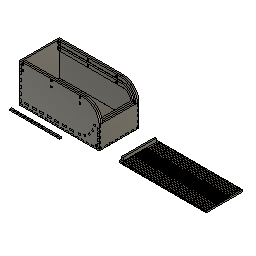
skuffa v30 (Autodesk Fusion 360 design; units mm, degrees)
Autodesk Fusion 360 part; units mm, degrees
note: some values were not read from the file. Chosen so that the rebuilt part matches the saved one: a direction. Set by a fixed rule: which sketch regions a step uses; which face or edge a step refers to.
(part 1 of 6)
sketch "Sketch1" plane through (0, 0, 0) normal (0, 0, 1) x (1, 0, 0)
  line L0 (2.6723, -62.3358) -> (29.1306, -62.3358)
  line L1 (29.1306, -62.3358) -> (29.1306, -59.69)
  line L2 (29.1306, -59.69) -> (2.6723, -59.69)
  line L3 (2.6723, -59.69) -> (2.6723, -62.3358)
  line L4 (5.3181, -57.2294) -> (4.5508, -57.2294)
  spline S0 degree 3 poles (4.5508, -57.2294) (4.5244, -57.2294) (4.5508, -57.2558) (4.5508, -57.2294) knots 0 0 0 0 1 1 1 1
  line L5 (4.5508, -57.2294) -> (4.5508, -56.4885)
  spline S1 degree 3 poles (4.5508, -56.4885) (4.5508, -56.4621) (4.5244, -56.4885) (4.5508, -56.4885) knots 0 0 0 0 1 1 1 1
  line L6 (4.5508, -56.4885) -> (6.0854, -56.4885)
  spline S2 degree 3 poles (6.0854, -56.4885) (6.1119, -56.4885) (6.0854, -56.4621) (6.0854, -56.4885) knots 0 0 0 0 1 1 1 1
  line L7 (6.0854, -56.4885) -> (6.0854, -57.2294)
  spline S3 degree 3 poles (6.0854, -57.2294) (6.0854, -57.2558) (6.1119, -57.2294) (6.0854, -57.2294) knots 0 0 0 0 1 1 1 1
  line L8 (6.0854, -57.2294) -> (5.3181, -57.2294)
  line L9 (8.4931, -57.2294) -> (7.7258, -57.2294)
  spline S4 degree 3 poles (7.7258, -57.2294) (7.6994, -57.2294) (7.7258, -57.2558) (7.7258, -57.2294) knots 0 0 0 0 1 1 1 1
  line L10 (7.7258, -57.2294) -> (7.7258, -56.4885)
  spline S5 degree 3 poles (7.7258, -56.4885) (7.7258, -56.4621) (7.6994, -56.4885) (7.7258, -56.4885) knots 0 0 0 0 1 1 1 1
  line L11 (7.7258, -56.4885) -> (9.2604, -56.4885)
  spline S6 degree 3 poles (9.2604, -56.4885) (9.2869, -56.4885) (9.2604, -56.4621) (9.2604, -56.4885) knots 0 0 0 0 1 1 1 1
  line L12 (9.2604, -56.4885) -> (9.2604, -57.2294)
  spline S7 degree 3 poles (9.2604, -57.2294) (9.2604, -57.2558) (9.2869, -57.2294) (9.2604, -57.2294) knots 0 0 0 0 1 1 1 1
  line L13 (9.2604, -57.2294) -> (8.4931, -57.2294)
  line L14 (11.6681, -57.2294) -> (10.9008, -57.2294)
  spline S8 degree 3 poles (10.9008, -57.2294) (10.8744, -57.2294) (10.9008, -57.2558) (10.9008, -57.2294) knots 0 0 0 0 1 1 1 1
  line L15 (10.9008, -57.2294) -> (10.9008, -56.4885)
  spline S9 degree 3 poles (10.9008, -56.4885) (10.9008, -56.4621) (10.8744, -56.4885) (10.9008, -56.4885) knots 0 0 0 0 1 1 1 1
  line L16 (10.9008, -56.4885) -> (12.4354, -56.4885)
  spline S10 degree 3 poles (12.4354, -56.4885) (12.4619, -56.4885) (12.4354, -56.4621) (12.4354, -56.4885) knots 0 0 0 0 1 1 1 1
  line L17 (12.4354, -56.4885) -> (12.4354, -57.2294)
  spline S11 degree 3 poles (12.4354, -57.2294) (12.4354, -57.2558) (12.4619, -57.2294) (12.4354, -57.2294) knots 0 0 0 0 1 1 1 1
  line L18 (12.4354, -57.2294) -> (11.6681, -57.2294)
  line L19 (14.8431, -57.2294) -> (14.0758, -57.2294)
  spline S12 degree 3 poles (14.0758, -57.2294) (14.0494, -57.2294) (14.0758, -57.2558) (14.0758, -57.2294) knots 0 0 0 0 1 1 1 1
  line L20 (14.0758, -57.2294) -> (14.0758, -56.4885)
  spline S13 degree 3 poles (14.0758, -56.4885) (14.0758, -56.4621) (14.0494, -56.4885) (14.0758, -56.4885) knots 0 0 0 0 1 1 1 1
  line L21 (14.0758, -56.4885) -> (15.6104, -56.4885)
  spline S14 degree 3 poles (15.6104, -56.4885) (15.6369, -56.4885) (15.6104, -56.4621) (15.6104, -56.4885) knots 0 0 0 0 1 1 1 1
  line L22 (15.6104, -56.4885) -> (15.6104, -57.2294)
  spline S15 degree 3 poles (15.6104, -57.2294) (15.6104, -57.2558) (15.6369, -57.2294) (15.6104, -57.2294) knots 0 0 0 0 1 1 1 1
  line L23 (15.6104, -57.2294) -> (14.8431, -57.2294)
  line L24 (18.0181, -57.2294) -> (17.2508, -57.2294)
  spline S16 degree 3 poles (17.2508, -57.2294) (17.2244, -57.2294) (17.2508, -57.2558) (17.2508, -57.2294) knots 0 0 0 0 1 1 1 1
  line L25 (17.2508, -57.2294) -> (17.2508, -56.4885)
  spline S17 degree 3 poles (17.2508, -56.4885) (17.2508, -56.4621) (17.2244, -56.4885) (17.2508, -56.4885) knots 0 0 0 0 1 1 1 1
  line L26 (17.2508, -56.4885) -> (18.7854, -56.4885)
  spline S18 degree 3 poles (18.7854, -56.4885) (18.8119, -56.4885) (18.7854, -56.4621) (18.7854, -56.4885) knots 0 0 0 0 1 1 1 1
  line L27 (18.7854, -56.4885) -> (18.7854, -57.2294)
  spline S19 degree 3 poles (18.7854, -57.2294) (18.7854, -57.2558) (18.8119, -57.2294) (18.7854, -57.2294) knots 0 0 0 0 1 1 1 1
  line L28 (18.7854, -57.2294) -> (18.0181, -57.2294)
  line L29 (21.1931, -57.2294) -> (20.4258, -57.2294)
  spline S20 degree 3 poles (20.4258, -57.2294) (20.3994, -57.2294) (20.4258, -57.2558) (20.4258, -57.2294) knots 0 0 0 0 1 1 1 1
  line L30 (20.4258, -57.2294) -> (20.4258, -56.4885)
  spline S21 degree 3 poles (20.4258, -56.4885) (20.4258, -56.4621) (20.3994, -56.4885) (20.4258, -56.4885) knots 0 0 0 0 1 1 1 1
  line L31 (20.4258, -56.4885) -> (21.9604, -56.4885)
  spline S22 degree 3 poles (21.9604, -56.4885) (21.9869, -56.4885) (21.9604, -56.4621) (21.9604, -56.4885) knots 0 0 0 0 1 1 1 1
  line L32 (21.9604, -56.4885) -> (21.9604, -57.2294)
  spline S23 degree 3 poles (21.9604, -57.2294) (21.9604, -57.2558) (21.9869, -57.2294) (21.9604, -57.2294) knots 0 0 0 0 1 1 1 1
  line L33 (21.9604, -57.2294) -> (21.1931, -57.2294)
  line L34 (24.3681, -57.2294) -> (23.6008, -57.2294)
  spline S24 degree 3 poles (23.6008, -57.2294) (23.5744, -57.2294) (23.6008, -57.2558) (23.6008, -57.2294) knots 0 0 0 0 1 1 1 1
  line L35 (23.6008, -57.2294) -> (23.6008, -56.4885)
  spline S25 degree 3 poles (23.6008, -56.4885) (23.6008, -56.4621) (23.5744, -56.4885) (23.6008, -56.4885) knots 0 0 0 0 1 1 1 1
  line L36 (23.6008, -56.4885) -> (25.1354, -56.4885)
  spline S26 degree 3 poles (25.1354, -56.4885) (25.1619, -56.4885) (25.1354, -56.4621) (25.1354, -56.4885) knots 0 0 0 0 1 1 1 1
  line L37 (25.1354, -56.4885) -> (25.1354, -57.2294)
  spline S27 degree 3 poles (25.1354, -57.2294) (25.1354, -57.2558) (25.1619, -57.2294) (25.1354, -57.2294) knots 0 0 0 0 1 1 1 1
  line L38 (25.1354, -57.2294) -> (24.3681, -57.2294)
  line L39 (27.5431, -57.2294) -> (26.7758, -57.2294)
  spline S28 degree 3 poles (26.7758, -57.2294) (26.7494, -57.2294) (26.7758, -57.2558) (26.7758, -57.2294) knots 0 0 0 0 1 1 1 1
  line L40 (26.7758, -57.2294) -> (26.7758, -56.4885)
  spline S29 degree 3 poles (26.7758, -56.4885) (26.7758, -56.4621) (26.7494, -56.4885) (26.7758, -56.4885) knots 0 0 0 0 1 1 1 1
  line L41 (26.7758, -56.4885) -> (28.3104, -56.4885)
  spline S30 degree 3 poles (28.3104, -56.4885) (28.3369, -56.4885) (28.3104, -56.4621) (28.3104, -56.4885) knots 0 0 0 0 1 1 1 1
  line L42 (28.3104, -56.4885) -> (28.3104, -57.2294)
  spline S31 degree 3 poles (28.3104, -57.2294) (28.3104, -57.2558) (28.3369, -57.2294) (28.3104, -57.2294) knots 0 0 0 0 1 1 1 1
  line L43 (28.3104, -57.2294) -> (27.5431, -57.2294)
  line L44 (30.7181, -57.2294) -> (29.9508, -57.2294)
  spline S32 degree 3 poles (29.9508, -57.2294) (29.9244, -57.2294) (29.9508, -57.2558) (29.9508, -57.2294) knots 0 0 0 0 1 1 1 1
  line L45 (29.9508, -57.2294) -> (29.9508, -56.4885)
  spline S33 degree 3 poles (29.9508, -56.4885) (29.9508, -56.4621) (29.9244, -56.4885) (29.9508, -56.4885) knots 0 0 0 0 1 1 1 1
  line L46 (29.9508, -56.4885) -> (31.4854, -56.4885)
  spline S34 degree 3 poles (31.4854, -56.4885) (31.5119, -56.4885) (31.4854, -56.4621) (31.4854, -56.4885) knots 0 0 0 0 1 1 1 1
  line L47 (31.4854, -56.4885) -> (31.4854, -57.2294)
  spline S35 degree 3 poles (31.4854, -57.2294) (31.4854, -57.2558) (31.5119, -57.2294) (31.4854, -57.2294) knots 0 0 0 0 1 1 1 1
  line L48 (31.4854, -57.2294) -> (30.7181, -57.2294)
  line L49 (34.9186, -56.6272) -> (34.1773, -56.8259)
  spline S36 degree 3 poles (34.1773, -56.8259) (34.1519, -56.8328) (34.1842, -56.8513) (34.1773, -56.8259) knots 0 0 0 0 1 1 1 1
  line L50 (34.1773, -56.8259) -> (33.9857, -56.1102)
  spline S37 degree 3 poles (33.9857, -56.1102) (33.9788, -56.0845) (33.9601, -56.1171) (33.9857, -56.1102) knots 0 0 0 0 1 1 1 1
  line L51 (33.9857, -56.1102) -> (35.4679, -55.713)
  spline S38 degree 3 poles (35.4679, -55.713) (35.4936, -55.7062) (35.461, -55.6874) (35.4679, -55.713) knots 0 0 0 0 1 1 1 1
  line L52 (35.4679, -55.713) -> (35.6597, -56.4287)
  spline S39 degree 3 poles (35.6597, -56.4287) (35.6666, -56.4541) (35.6851, -56.4219) (35.6597, -56.4287) knots 0 0 0 0 1 1 1 1
  line L53 (35.6597, -56.4287) -> (34.9186, -56.6272)
  line L54 (38.9861, -54.279) -> (38.4434, -54.8214)
  spline S40 degree 3 poles (38.4434, -54.8214) (38.4246, -54.8402) (38.4622, -54.8402) (38.4434, -54.8214) knots 0 0 0 0 1 1 1 1
  line L55 (38.4434, -54.8214) -> (37.9196, -54.2975)
  spline S41 degree 3 poles (37.9196, -54.2975) (37.9008, -54.279) (37.9008, -54.3163) (37.9196, -54.2975) knots 0 0 0 0 1 1 1 1
  line L56 (37.9196, -54.2975) -> (39.0046, -53.2125)
  spline S42 degree 3 poles (39.0046, -53.2125) (39.0234, -53.1937) (38.9861, -53.1937) (39.0046, -53.2125) knots 0 0 0 0 1 1 1 1
  line L57 (39.0046, -53.2125) -> (39.5285, -53.7363)
  spline S43 degree 3 poles (39.5285, -53.7363) (39.5473, -53.7551) (39.5473, -53.7176) (39.5285, -53.7363) knots 0 0 0 0 1 1 1 1
  line L58 (39.5285, -53.7363) -> (38.9861, -54.279)
  line L59 (41.3343, -50.2116) -> (41.1358, -50.9527)
  spline S44 degree 3 poles (41.1358, -50.9527) (41.1289, -50.9781) (41.1612, -50.9595) (41.1358, -50.9527) knots 0 0 0 0 1 1 1 1
  line L60 (41.1358, -50.9527) -> (40.4201, -50.7608)
  spline S45 degree 3 poles (40.4201, -50.7608) (40.3945, -50.754) (40.4133, -50.7865) (40.4201, -50.7608) knots 0 0 0 0 1 1 1 1
  line L61 (40.4201, -50.7608) -> (40.8173, -49.2786)
  spline S46 degree 3 poles (40.8173, -49.2786) (40.8242, -49.253) (40.7916, -49.2718) (40.8173, -49.2786) knots 0 0 0 0 1 1 1 1
  line L62 (40.8173, -49.2786) -> (41.533, -49.4702)
  spline S47 degree 3 poles (41.533, -49.4702) (41.5584, -49.4771) (41.5398, -49.4448) (41.533, -49.4702) knots 0 0 0 0 1 1 1 1
  line L63 (41.533, -49.4702) -> (41.3343, -50.2116)
  line L64 (41.9365, -45.2173) -> (41.9365, -45.9846)
  spline S48 degree 3 poles (41.9365, -45.9846) (41.9365, -46.011) (41.9629, -45.9846) (41.9365, -45.9846) knots 0 0 0 0 1 1 1 1
  line L65 (41.9365, -45.9846) -> (41.1956, -45.9846)
  spline S49 degree 3 poles (41.1956, -45.9846) (41.1692, -45.9846) (41.1956, -46.011) (41.1956, -45.9846) knots 0 0 0 0 1 1 1 1
  line L66 (41.1956, -45.9846) -> (41.1956, -44.45)
  spline S50 degree 3 poles (41.1956, -44.45) (41.1956, -44.4235) (41.1692, -44.45) (41.1956, -44.45) knots 0 0 0 0 1 1 1 1
  line L67 (41.1956, -44.45) -> (41.9365, -44.45)
  spline S51 degree 3 poles (41.9365, -44.45) (41.9629, -44.45) (41.9365, -44.4235) (41.9365, -44.45) knots 0 0 0 0 1 1 1 1
  line L68 (41.9365, -44.45) -> (41.9365, -45.2173)
  line L69 (3.466, -58.4465) -> (5.0271, -58.4465)
  spline S52 degree 3 poles (5.0271, -58.4465) (5.0535, -58.4465) (5.0271, -58.42) (5.0271, -58.4465) knots 0 0 0 0 1 1 1 1
  line L70 (5.0271, -58.4465) -> (5.0271, -59.2138)
  spline S53 degree 3 poles (5.0271, -59.2138) (5.0271, -59.2283) (5.039, -59.2402) (5.0535, -59.2402) knots 0 0 0 0 1 1 1 1
  line L71 (5.0535, -59.2402) -> (6.641, -59.2402)
  spline S54 degree 3 poles (6.641, -59.2402) (6.6556, -59.2402) (6.6675, -59.2283) (6.6675, -59.2138) knots 0 0 0 0 1 1 1 1
  line L72 (6.6675, -59.2138) -> (6.6675, -58.4465)
  spline S55 degree 3 poles (6.6675, -58.4465) (6.6675, -58.42) (6.641, -58.4465) (6.6675, -58.4465) knots 0 0 0 0 1 1 1 1
  line L73 (6.6675, -58.4465) -> (8.2021, -58.4465)
  spline S56 degree 3 poles (8.2021, -58.4465) (8.2285, -58.4465) (8.2021, -58.42) (8.2021, -58.4465) knots 0 0 0 0 1 1 1 1
  line L74 (8.2021, -58.4465) -> (8.2021, -59.2138)
  spline S57 degree 3 poles (8.2021, -59.2138) (8.2021, -59.2283) (8.214, -59.2402) (8.2285, -59.2402) knots 0 0 0 0 1 1 1 1
  line L75 (8.2285, -59.2402) -> (9.816, -59.2402)
  spline S58 degree 3 poles (9.816, -59.2402) (9.8306, -59.2402) (9.8425, -59.2283) (9.8425, -59.2138) knots 0 0 0 0 1 1 1 1
  line L76 (9.8425, -59.2138) -> (9.8425, -58.4465)
  spline S59 degree 3 poles (9.8425, -58.4465) (9.8425, -58.42) (9.816, -58.4465) (9.8425, -58.4465) knots 0 0 0 0 1 1 1 1
  line L77 (9.8425, -58.4465) -> (11.3771, -58.4465)
  spline S60 degree 3 poles (11.3771, -58.4465) (11.4035, -58.4465) (11.3771, -58.42) (11.3771, -58.4465) knots 0 0 0 0 1 1 1 1
  line L78 (11.3771, -58.4465) -> (11.3771, -59.2138)
  spline S61 degree 3 poles (11.3771, -59.2138) (11.3771, -59.2283) (11.389, -59.2402) (11.4035, -59.2402) knots 0 0 0 0 1 1 1 1
  line L79 (11.4035, -59.2402) -> (12.991, -59.2402)
  spline S62 degree 3 poles (12.991, -59.2402) (13.0056, -59.2402) (13.0175, -59.2283) (13.0175, -59.2138) knots 0 0 0 0 1 1 1 1
  line L80 (13.0175, -59.2138) -> (13.0175, -58.4465)
  spline S63 degree 3 poles (13.0175, -58.4465) (13.0175, -58.42) (12.991, -58.4465) (13.0175, -58.4465) knots 0 0 0 0 1 1 1 1
  line L81 (13.0175, -58.4465) -> (14.5521, -58.4465)
  spline S64 degree 3 poles (14.5521, -58.4465) (14.5785, -58.4465) (14.5521, -58.42) (14.5521, -58.4465) knots 0 0 0 0 1 1 1 1
  line L82 (14.5521, -58.4465) -> (14.5521, -59.2138)
  spline S65 degree 3 poles (14.5521, -59.2138) (14.5521, -59.2283) (14.564, -59.2402) (14.5785, -59.2402) knots 0 0 0 0 1 1 1 1
  line L83 (14.5785, -59.2402) -> (16.166, -59.2402)
  spline S66 degree 3 poles (16.166, -59.2402) (16.1806, -59.2402) (16.1925, -59.2283) (16.1925, -59.2138) knots 0 0 0 0 1 1 1 1
  line L84 (16.1925, -59.2138) -> (16.1925, -58.4465)
  spline S67 degree 3 poles (16.1925, -58.4465) (16.1925, -58.42) (16.166, -58.4465) (16.1925, -58.4465) knots 0 0 0 0 1 1 1 1
  line L85 (16.1925, -58.4465) -> (17.7271, -58.4465)
  spline S68 degree 3 poles (17.7271, -58.4465) (17.7535, -58.4465) (17.7271, -58.42) (17.7271, -58.4465) knots 0 0 0 0 1 1 1 1
  line L86 (17.7271, -58.4465) -> (17.7271, -59.2138)
  spline S69 degree 3 poles (17.7271, -59.2138) (17.7271, -59.2283) (17.739, -59.2402) (17.7535, -59.2402) knots 0 0 0 0 1 1 1 1
  line L87 (17.7535, -59.2402) -> (19.341, -59.2402)
  spline S70 degree 3 poles (19.341, -59.2402) (19.3556, -59.2402) (19.3675, -59.2283) (19.3675, -59.2138) knots 0 0 0 0 1 1 1 1
  line L88 (19.3675, -59.2138) -> (19.3675, -58.4465)
  spline S71 degree 3 poles (19.3675, -58.4465) (19.3675, -58.42) (19.341, -58.4465) (19.3675, -58.4465) knots 0 0 0 0 1 1 1 1
  line L89 (19.3675, -58.4465) -> (20.9021, -58.4465)
  spline S72 degree 3 poles (20.9021, -58.4465) (20.9285, -58.4465) (20.9021, -58.42) (20.9021, -58.4465) knots 0 0 0 0 1 1 1 1
  line L90 (20.9021, -58.4465) -> (20.9021, -59.2138)
  spline S73 degree 3 poles (20.9021, -59.2138) (20.9021, -59.2283) (20.914, -59.2402) (20.9285, -59.2402) knots 0 0 0 0 1 1 1 1
  line L91 (20.9285, -59.2402) -> (22.516, -59.2402)
  spline S74 degree 3 poles (22.516, -59.2402) (22.5306, -59.2402) (22.5425, -59.2283) (22.5425, -59.2138) knots 0 0 0 0 1 1 1 1
  line L92 (22.5425, -59.2138) -> (22.5425, -58.4465)
  spline S75 degree 3 poles (22.5425, -58.4465) (22.5425, -58.42) (22.516, -58.4465) (22.5425, -58.4465) knots 0 0 0 0 1 1 1 1
  line L93 (22.5425, -58.4465) -> (24.0771, -58.4465)
  spline S76 degree 3 poles (24.0771, -58.4465) (24.1035, -58.4465) (24.0771, -58.42) (24.0771, -58.4465) knots 0 0 0 0 1 1 1 1
  line L94 (24.0771, -58.4465) -> (24.0771, -59.2138)
  spline S77 degree 3 poles (24.0771, -59.2138) (24.0771, -59.2283) (24.089, -59.2402) (24.1035, -59.2402) knots 0 0 0 0 1 1 1 1
  line L95 (24.1035, -59.2402) -> (25.691, -59.2402)
  spline S78 degree 3 poles (25.691, -59.2402) (25.7056, -59.2402) (25.7175, -59.2283) (25.7175, -59.2138) knots 0 0 0 0 1 1 1 1
  line L96 (25.7175, -59.2138) -> (25.7175, -58.4465)
  spline S79 degree 3 poles (25.7175, -58.4465) (25.7175, -58.42) (25.691, -58.4465) (25.7175, -58.4465) knots 0 0 0 0 1 1 1 1
  line L97 (25.7175, -58.4465) -> (27.2521, -58.4465)
  spline S80 degree 3 poles (27.2521, -58.4465) (27.2785, -58.4465) (27.2521, -58.42) (27.2521, -58.4465) knots 0 0 0 0 1 1 1 1
  line L98 (27.2521, -58.4465) -> (27.2521, -59.2138)
  spline S81 degree 3 poles (27.2521, -59.2138) (27.2521, -59.2283) (27.264, -59.2402) (27.2785, -59.2402) knots 0 0 0 0 1 1 1 1
  line L99 (27.2785, -59.2402) -> (28.866, -59.2402)
  spline S82 degree 3 poles (28.866, -59.2402) (28.8806, -59.2402) (28.8925, -59.2283) (28.8925, -59.2138) knots 0 0 0 0 1 1 1 1
  line L100 (28.8925, -59.2138) -> (28.8925, -58.4465)
  spline S83 degree 3 poles (28.8925, -58.4465) (28.8925, -58.42) (28.866, -58.4465) (28.8925, -58.4465) knots 0 0 0 0 1 1 1 1
  line L101 (28.8925, -58.4465) -> (30.4271, -58.4465)
  spline S84 degree 3 poles (30.4271, -58.4465) (30.4535, -58.4465) (30.4271, -58.42) (30.4271, -58.4465) knots 0 0 0 0 1 1 1 1
  line L102 (30.4271, -58.4465) -> (30.4271, -59.2138)
  spline S85 degree 3 poles (30.4271, -59.2138) (30.4271, -59.2283) (30.439, -59.2402) (30.4535, -59.2402) knots 0 0 0 0 1 1 1 1
  line L103 (30.4535, -59.2402) -> (32.041, -59.2402)
  spline S86 degree 3 poles (32.041, -59.2402) (32.0556, -59.2402) (32.0675, -59.2283) (32.0675, -59.2138) knots 0 0 0 0 1 1 1 1
  line L104 (32.0675, -59.2138) -> (32.0675, -58.4465)
  spline S87 degree 3 poles (32.0675, -58.4465) (32.0675, -58.42) (32.041, -58.4465) (32.0675, -58.4465) knots 0 0 0 0 1 1 1 1
  line L105 (32.0675, -58.4465) -> (33.6021, -58.4465)
  spline S88 degree 3 poles (33.6021, -58.4465) (33.6285, -58.4465) (33.6021, -58.42) (33.6021, -58.4465) knots 0 0 0 0 1 1 1 1
  line L106 (33.6021, -58.4465) -> (33.6021, -59.2138)
  spline S89 degree 3 poles (33.6021, -59.2138) (33.6021, -59.2283) (33.614, -59.2402) (33.6285, -59.2402) knots 0 0 0 0 1 1 1 1
  line L107 (33.6285, -59.2402) -> (35.216, -59.2402)
  spline S90 degree 3 poles (35.216, -59.2402) (35.2306, -59.2402) (35.2425, -59.2283) (35.2425, -59.2138) knots 0 0 0 0 1 1 1 1
  line L108 (35.2425, -59.2138) -> (35.2425, -58.4465)
  spline S91 degree 3 poles (35.2425, -58.4465) (35.2425, -58.42) (35.216, -58.4465) (35.2425, -58.4465) knots 0 0 0 0 1 1 1 1
  line L109 (35.2425, -58.4465) -> (36.7771, -58.4465)
  spline S92 degree 3 poles (36.7771, -58.4465) (36.8035, -58.4465) (36.7771, -58.42) (36.7771, -58.4465) knots 0 0 0 0 1 1 1 1
  line L110 (36.7771, -58.4465) -> (36.7771, -59.2138)
  spline S93 degree 3 poles (36.7771, -59.2138) (36.7771, -59.2283) (36.789, -59.2402) (36.8035, -59.2402) knots 0 0 0 0 1 1 1 1
  line L111 (36.8035, -59.2402) -> (38.391, -59.2402)
  spline S94 degree 3 poles (38.391, -59.2402) (38.4056, -59.2402) (38.4175, -59.2283) (38.4175, -59.2138) knots 0 0 0 0 1 1 1 1
  line L112 (38.4175, -59.2138) -> (38.4175, -58.4465)
  spline S95 degree 3 poles (38.4175, -58.4465) (38.4175, -58.42) (38.391, -58.4465) (38.4175, -58.4465) knots 0 0 0 0 1 1 1 1
  line L113 (38.4175, -58.4465) -> (39.9521, -58.4465)
  spline S96 degree 3 poles (39.9521, -58.4465) (39.9785, -58.4465) (39.9521, -58.42) (39.9521, -58.4465) knots 0 0 0 0 1 1 1 1
  line L114 (39.9521, -58.4465) -> (39.9521, -59.2138)
  spline S97 degree 3 poles (39.9521, -59.2138) (39.9521, -59.2283) (39.964, -59.2402) (39.9785, -59.2402) knots 0 0 0 0 1 1 1 1
  line L115 (39.9785, -59.2402) -> (41.566, -59.2402)
  spline S98 degree 3 poles (41.566, -59.2402) (41.5806, -59.2402) (41.5925, -59.2283) (41.5925, -59.2138) knots 0 0 0 0 1 1 1 1
  line L116 (41.5925, -59.2138) -> (41.5925, -58.4465)
  spline S99 degree 3 poles (41.5925, -58.4465) (41.5925, -58.42) (41.566, -58.4465) (41.5925, -58.4465) knots 0 0 0 0 1 1 1 1
  line L117 (41.5925, -58.4465) -> (43.1535, -58.4465)
  spline S100 degree 3 poles (43.1535, -58.4465) (43.1681, -58.4465) (43.18, -58.4346) (43.18, -58.42) knots 0 0 0 0 1 1 1 1
  line L118 (43.18, -58.42) -> (43.18, -57.6527)
  spline S101 degree 3 poles (43.18, -57.6527) (43.18, -57.6263) (43.1535, -57.6527) (43.18, -57.6527) knots 0 0 0 0 1 1 1 1
  line L119 (43.18, -57.6527) -> (43.9473, -57.6527)
  spline S102 degree 3 poles (43.9473, -57.6527) (43.9618, -57.6527) (43.9737, -57.6408) (43.9737, -57.6263) knots 0 0 0 0 1 1 1 1
  line L120 (43.9737, -57.6263) -> (43.9737, -56.0388)
  spline S103 degree 3 poles (43.9737, -56.0388) (43.9737, -56.0242) (43.9618, -56.0123) (43.9473, -56.0123) knots 0 0 0 0 1 1 1 1
  line L121 (43.9473, -56.0123) -> (43.18, -56.0123)
  spline S104 degree 3 poles (43.18, -56.0123) (43.1535, -56.0123) (43.18, -56.0388) (43.18, -56.0123) knots 0 0 0 0 1 1 1 1
  line L122 (43.18, -56.0123) -> (43.18, -54.4777)
  spline S105 degree 3 poles (43.18, -54.4777) (43.18, -54.4513) (43.1535, -54.4777) (43.18, -54.4777) knots 0 0 0 0 1 1 1 1
  line L123 (43.18, -54.4777) -> (43.9473, -54.4777)
  spline S106 degree 3 poles (43.9473, -54.4777) (43.9618, -54.4777) (43.9737, -54.4658) (43.9737, -54.4513) knots 0 0 0 0 1 1 1 1
  line L124 (43.9737, -54.4513) -> (43.9737, -52.8638)
  spline S107 degree 3 poles (43.9737, -52.8638) (43.9737, -52.8492) (43.9618, -52.8373) (43.9473, -52.8373) knots 0 0 0 0 1 1 1 1
  line L125 (43.9473, -52.8373) -> (43.18, -52.8373)
  spline S108 degree 3 poles (43.18, -52.8373) (43.1535, -52.8373) (43.18, -52.8638) (43.18, -52.8373) knots 0 0 0 0 1 1 1 1
  line L126 (43.18, -52.8373) -> (43.18, -51.3027)
  spline S109 degree 3 poles (43.18, -51.3027) (43.18, -51.2763) (43.1535, -51.3027) (43.18, -51.3027) knots 0 0 0 0 1 1 1 1
  line L127 (43.18, -51.3027) -> (43.9473, -51.3027)
  spline S110 degree 3 poles (43.9473, -51.3027) (43.9618, -51.3027) (43.9737, -51.2908) (43.9737, -51.2763) knots 0 0 0 0 1 1 1 1
  line L128 (43.9737, -51.2763) -> (43.9737, -49.6888)
  spline S111 degree 3 poles (43.9737, -49.6888) (43.9737, -49.6742) (43.9618, -49.6623) (43.9473, -49.6623) knots 0 0 0 0 1 1 1 1
  line L129 (43.9473, -49.6623) -> (43.18, -49.6623)
  spline S112 degree 3 poles (43.18, -49.6623) (43.1535, -49.6623) (43.18, -49.6888) (43.18, -49.6623) knots 0 0 0 0 1 1 1 1
  line L130 (43.18, -49.6623) -> (43.18, -48.1277)
  spline S113 degree 3 poles (43.18, -48.1277) (43.18, -48.1013) (43.1535, -48.1277) (43.18, -48.1277) knots 0 0 0 0 1 1 1 1
  line L131 (43.18, -48.1277) -> (43.9473, -48.1277)
  spline S114 degree 3 poles (43.9473, -48.1277) (43.9618, -48.1277) (43.9737, -48.1158) (43.9737, -48.1013) knots 0 0 0 0 1 1 1 1
  line L132 (43.9737, -48.1013) -> (43.9737, -46.5138)
  spline S115 degree 3 poles (43.9737, -46.5138) (43.9737, -46.4992) (43.9618, -46.4873) (43.9473, -46.4873) knots 0 0 0 0 1 1 1 1
  line L133 (43.9473, -46.4873) -> (43.18, -46.4873)
  spline S116 degree 3 poles (43.18, -46.4873) (43.1535, -46.4873) (43.18, -46.5138) (43.18, -46.4873) knots 0 0 0 0 1 1 1 1
  line L134 (43.18, -46.4873) -> (43.18, -44.9527)
  spline S117 degree 3 poles (43.18, -44.9527) (43.18, -44.9263) (43.1535, -44.9527) (43.18, -44.9527) knots 0 0 0 0 1 1 1 1
  line L135 (43.18, -44.9527) -> (43.9473, -44.9527)
  spline S118 degree 3 poles (43.9473, -44.9527) (43.9618, -44.9527) (43.9737, -44.9408) (43.9737, -44.9263) knots 0 0 0 0 1 1 1 1
  line L136 (43.9737, -44.9263) -> (43.9737, -43.3388)
  spline S119 degree 3 poles (43.9737, -43.3388) (43.9737, -43.3242) (43.9618, -43.3123) (43.9473, -43.3123) knots 0 0 0 0 1 1 1 1
  line L137 (43.9473, -43.3123) -> (43.18, -43.3123)
  spline S120 degree 3 poles (43.18, -43.3123) (43.1535, -43.3123) (43.18, -43.3388) (43.18, -43.3123) knots 0 0 0 0 1 1 1 1
  line L138 (43.18, -43.3123) -> (43.18, -42.5715)
  spline S121 degree 3 poles (43.18, -42.5715) (43.18, -42.545) (43.1535, -42.5715) (43.18, -42.5715) knots 0 0 0 0 1 1 1 1
  line L139 (43.18, -42.5715) -> (43.9473, -42.5715)
  spline S122 degree 3 poles (43.9473, -42.5715) (43.9618, -42.5715) (43.9737, -42.5596) (43.9737, -42.545) knots 0 0 0 0 1 1 1 1
  spline S123 degree 3 poles (43.9737, -42.545) (43.9737, -40.5432) (43.447, -38.5768) (42.446, -36.8432) knots 0 0 0 0 1 1 1 1
  spline S124 degree 3 poles (42.446, -36.8432) (41.4451, -35.1097) (40.0055, -33.6701) (38.272, -32.6692) knots 0 0 0 0 1 1 1 1
  spline S125 degree 3 poles (38.272, -32.6692) (36.5384, -31.6682) (34.572, -31.1415) (32.5702, -31.1415) knots 0 0 0 0 1 1 1 1
  line L140 (32.5702, -31.1415) -> (3.466, -31.1415)
  spline S126 degree 3 poles (3.466, -31.1415) (3.4515, -31.1415) (3.4396, -31.1534) (3.4396, -31.1679) knots 0 0 0 0 1 1 1 1
  line L141 (3.4396, -31.1679) -> (3.4396, -31.9617)
  line L142 (3.4396, -31.9617) -> (3.4396, -33.2581)
  spline S127 degree 3 poles (3.4396, -33.2581) (3.4396, -33.2846) (3.466, -33.2581) (3.4396, -33.2581) knots 0 0 0 0 1 1 1 1
  line L143 (3.4396, -33.2581) -> (2.6723, -33.2581)
  spline S128 degree 3 poles (2.6723, -33.2581) (2.6577, -33.2581) (2.6458, -33.27) (2.6458, -33.2846) knots 0 0 0 0 1 1 1 1
  line L144 (2.6458, -33.2846) -> (2.6458, -34.8721)
  spline S129 degree 3 poles (2.6458, -34.8721) (2.6458, -34.8866) (2.6577, -34.8985) (2.6723, -34.8985) knots 0 0 0 0 1 1 1 1
  line L145 (2.6723, -34.8985) -> (3.4396, -34.8985)
  spline S130 degree 3 poles (3.4396, -34.8985) (3.466, -34.8985) (3.4396, -34.8721) (3.4396, -34.8985) knots 0 0 0 0 1 1 1 1
  line L146 (3.4396, -34.8985) -> (3.4396, -36.4331)
  spline S131 degree 3 poles (3.4396, -36.4331) (3.4396, -36.4596) (3.466, -36.4331) (3.4396, -36.4331) knots 0 0 0 0 1 1 1 1
  line L147 (3.4396, -36.4331) -> (2.6723, -36.4331)
  spline S132 degree 3 poles (2.6723, -36.4331) (2.6577, -36.4331) (2.6458, -36.445) (2.6458, -36.4596) knots 0 0 0 0 1 1 1 1
  line L148 (2.6458, -36.4596) -> (2.6458, -38.0471)
  spline S133 degree 3 poles (2.6458, -38.0471) (2.6458, -38.0616) (2.6577, -38.0735) (2.6723, -38.0735) knots 0 0 0 0 1 1 1 1
  line L149 (2.6723, -38.0735) -> (3.4396, -38.0735)
  spline S134 degree 3 poles (3.4396, -38.0735) (3.466, -38.0735) (3.4396, -38.0471) (3.4396, -38.0735) knots 0 0 0 0 1 1 1 1
  line L150 (3.4396, -38.0735) -> (3.4396, -39.6081)
  spline S135 degree 3 poles (3.4396, -39.6081) (3.4396, -39.6346) (3.466, -39.6081) (3.4396, -39.6081) knots 0 0 0 0 1 1 1 1
  line L151 (3.4396, -39.6081) -> (2.6723, -39.6081)
  spline S136 degree 3 poles (2.6723, -39.6081) (2.6577, -39.6081) (2.6458, -39.62) (2.6458, -39.6346) knots 0 0 0 0 1 1 1 1
  line L152 (2.6458, -39.6346) -> (2.6458, -41.2221)
  spline S137 degree 3 poles (2.6458, -41.2221) (2.6458, -41.2366) (2.6577, -41.2485) (2.6723, -41.2485) knots 0 0 0 0 1 1 1 1
  line L153 (2.6723, -41.2485) -> (3.4396, -41.2485)
  spline S138 degree 3 poles (3.4396, -41.2485) (3.466, -41.2485) (3.4396, -41.2221) (3.4396, -41.2485) knots 0 0 0 0 1 1 1 1
  line L154 (3.4396, -41.2485) -> (3.4396, -42.7831)
  spline S139 degree 3 poles (3.4396, -42.7831) (3.4396, -42.8096) (3.466, -42.7831) (3.4396, -42.7831) knots 0 0 0 0 1 1 1 1
  line L155 (3.4396, -42.7831) -> (2.6723, -42.7831)
  spline S140 degree 3 poles (2.6723, -42.7831) (2.6577, -42.7831) (2.6458, -42.795) (2.6458, -42.8096) knots 0 0 0 0 1 1 1 1
  line L156 (2.6458, -42.8096) -> (2.6458, -44.3971)
  spline S141 degree 3 poles (2.6458, -44.3971) (2.6458, -44.4116) (2.6577, -44.4235) (2.6723, -44.4235) knots 0 0 0 0 1 1 1 1
  line L157 (2.6723, -44.4235) -> (3.4396, -44.4235)
  spline S142 degree 3 poles (3.4396, -44.4235) (3.466, -44.4235) (3.4396, -44.3971) (3.4396, -44.4235) knots 0 0 0 0 1 1 1 1
  line L158 (3.4396, -44.4235) -> (3.4396, -45.9581)
  spline S143 degree 3 poles (3.4396, -45.9581) (3.4396, -45.9846) (3.466, -45.9581) (3.4396, -45.9581) knots 0 0 0 0 1 1 1 1
  line L159 (3.4396, -45.9581) -> (2.6723, -45.9581)
  spline S144 degree 3 poles (2.6723, -45.9581) (2.6577, -45.9581) (2.6458, -45.97) (2.6458, -45.9846) knots 0 0 0 0 1 1 1 1
  line L160 (2.6458, -45.9846) -> (2.6458, -47.5721)
  spline S145 degree 3 poles (2.6458, -47.5721) (2.6458, -47.5866) (2.6577, -47.5985) (2.6723, -47.5985) knots 0 0 0 0 1 1 1 1
  line L161 (2.6723, -47.5985) -> (3.4396, -47.5985)
  spline S146 degree 3 poles (3.4396, -47.5985) (3.466, -47.5985) (3.4396, -47.5721) (3.4396, -47.5985) knots 0 0 0 0 1 1 1 1
  line L162 (3.4396, -47.5985) -> (3.4396, -49.1331)
  spline S147 degree 3 poles (3.4396, -49.1331) (3.4396, -49.1596) (3.466, -49.1331) (3.4396, -49.1331) knots 0 0 0 0 1 1 1 1
  line L163 (3.4396, -49.1331) -> (2.6723, -49.1331)
  spline S148 degree 3 poles (2.6723, -49.1331) (2.6577, -49.1331) (2.6458, -49.145) (2.6458, -49.1596) knots 0 0 0 0 1 1 1 1
  line L164 (2.6458, -49.1596) -> (2.6458, -50.7471)
  spline S149 degree 3 poles (2.6458, -50.7471) (2.6458, -50.7616) (2.6577, -50.7735) (2.6723, -50.7735) knots 0 0 0 0 1 1 1 1
  line L165 (2.6723, -50.7735) -> (3.4396, -50.7735)
  spline S150 degree 3 poles (3.4396, -50.7735) (3.466, -50.7735) (3.4396, -50.7471) (3.4396, -50.7735) knots 0 0 0 0 1 1 1 1
  line L166 (3.4396, -50.7735) -> (3.4396, -52.3081)
  spline S151 degree 3 poles (3.4396, -52.3081) (3.4396, -52.3346) (3.466, -52.3081) (3.4396, -52.3081) knots 0 0 0 0 1 1 1 1
  line L167 (3.4396, -52.3081) -> (2.6723, -52.3081)
  spline S152 degree 3 poles (2.6723, -52.3081) (2.6577, -52.3081) (2.6458, -52.32) (2.6458, -52.3346) knots 0 0 0 0 1 1 1 1
  line L168 (2.6458, -52.3346) -> (2.6458, -53.9221)
  spline S153 degree 3 poles (2.6458, -53.9221) (2.6458, -53.9366) (2.6577, -53.9485) (2.6723, -53.9485) knots 0 0 0 0 1 1 1 1
  line L169 (2.6723, -53.9485) -> (3.4396, -53.9485)
  spline S154 degree 3 poles (3.4396, -53.9485) (3.466, -53.9485) (3.4396, -53.9221) (3.4396, -53.9485) knots 0 0 0 0 1 1 1 1
  line L170 (3.4396, -53.9485) -> (3.4396, -55.4831)
  spline S155 degree 3 poles (3.4396, -55.4831) (3.4396, -55.5096) (3.466, -55.4831) (3.4396, -55.4831) knots 0 0 0 0 1 1 1 1
  line L171 (3.4396, -55.4831) -> (2.6723, -55.4831)
  spline S156 degree 3 poles (2.6723, -55.4831) (2.6577, -55.4831) (2.6458, -55.495) (2.6458, -55.5096) knots 0 0 0 0 1 1 1 1
  line L172 (2.6458, -55.5096) -> (2.6458, -57.0971)
  spline S157 degree 3 poles (2.6458, -57.0971) (2.6458, -57.1116) (2.6577, -57.1235) (2.6723, -57.1235) knots 0 0 0 0 1 1 1 1
  line L173 (2.6723, -57.1235) -> (3.4396, -57.1235)
  spline S158 degree 3 poles (3.4396, -57.1235) (3.466, -57.1235) (3.4396, -57.0971) (3.4396, -57.1235) knots 0 0 0 0 1 1 1 1
  line L174 (3.4396, -57.1235) -> (3.4396, -58.42)
  line L175 (47.0429, -57.2294) -> (46.2756, -57.2294)
  spline S159 degree 3 poles (46.2756, -57.2294) (46.2492, -57.2294) (46.2756, -57.2558) (46.2756, -57.2294) knots 0 0 0 0 1 1 1 1
  line L176 (46.2756, -57.2294) -> (46.2756, -56.4885)
  spline S160 degree 3 poles (46.2756, -56.4885) (46.2756, -56.4621) (46.2492, -56.4885) (46.2756, -56.4885) knots 0 0 0 0 1 1 1 1
  line L177 (46.2756, -56.4885) -> (47.8102, -56.4885)
  spline S161 degree 3 poles (47.8102, -56.4885) (47.8367, -56.4885) (47.8102, -56.4621) (47.8102, -56.4885) knots 0 0 0 0 1 1 1 1
  line L178 (47.8102, -56.4885) -> (47.8102, -57.2294)
  spline S162 degree 3 poles (47.8102, -57.2294) (47.8102, -57.2558) (47.8367, -57.2294) (47.8102, -57.2294) knots 0 0 0 0 1 1 1 1
  line L179 (47.8102, -57.2294) -> (47.0429, -57.2294)
  line L180 (50.2179, -57.2294) -> (49.4506, -57.2294)
  spline S163 degree 3 poles (49.4506, -57.2294) (49.4242, -57.2294) (49.4506, -57.2558) (49.4506, -57.2294) knots 0 0 0 0 1 1 1 1
  line L181 (49.4506, -57.2294) -> (49.4506, -56.4885)
  spline S164 degree 3 poles (49.4506, -56.4885) (49.4506, -56.4621) (49.4242, -56.4885) (49.4506, -56.4885) knots 0 0 0 0 1 1 1 1
  line L182 (49.4506, -56.4885) -> (50.9852, -56.4885)
  spline S165 degree 3 poles (50.9852, -56.4885) (51.0117, -56.4885) (50.9852, -56.4621) (50.9852, -56.4885) knots 0 0 0 0 1 1 1 1
  line L183 (50.9852, -56.4885) -> (50.9852, -57.2294)
  spline S166 degree 3 poles (50.9852, -57.2294) (50.9852, -57.2558) (51.0117, -57.2294) (50.9852, -57.2294) knots 0 0 0 0 1 1 1 1
  line L184 (50.9852, -57.2294) -> (50.2179, -57.2294)
  line L185 (53.3929, -57.2294) -> (52.6256, -57.2294)
  spline S167 degree 3 poles (52.6256, -57.2294) (52.5992, -57.2294) (52.6256, -57.2558) (52.6256, -57.2294) knots 0 0 0 0 1 1 1 1
  line L186 (52.6256, -57.2294) -> (52.6256, -56.4885)
  spline S168 degree 3 poles (52.6256, -56.4885) (52.6256, -56.4621) (52.5992, -56.4885) (52.6256, -56.4885) knots 0 0 0 0 1 1 1 1
  line L187 (52.6256, -56.4885) -> (54.1602, -56.4885)
  spline S169 degree 3 poles (54.1602, -56.4885) (54.1867, -56.4885) (54.1602, -56.4621) (54.1602, -56.4885) knots 0 0 0 0 1 1 1 1
  line L188 (54.1602, -56.4885) -> (54.1602, -57.2294)
  spline S170 degree 3 poles (54.1602, -57.2294) (54.1602, -57.2558) (54.1867, -57.2294) (54.1602, -57.2294) knots 0 0 0 0 1 1 1 1
  line L189 (54.1602, -57.2294) -> (53.3929, -57.2294)
  line L190 (56.5679, -57.2294) -> (55.8006, -57.2294)
  spline S171 degree 3 poles (55.8006, -57.2294) (55.7742, -57.2294) (55.8006, -57.2558) (55.8006, -57.2294) knots 0 0 0 0 1 1 1 1
  line L191 (55.8006, -57.2294) -> (55.8006, -56.4885)
  spline S172 degree 3 poles (55.8006, -56.4885) (55.8006, -56.4621) (55.7742, -56.4885) (55.8006, -56.4885) knots 0 0 0 0 1 1 1 1
  line L192 (55.8006, -56.4885) -> (57.3352, -56.4885)
  spline S173 degree 3 poles (57.3352, -56.4885) (57.3617, -56.4885) (57.3352, -56.4621) (57.3352, -56.4885) knots 0 0 0 0 1 1 1 1
  line L193 (57.3352, -56.4885) -> (57.3352, -57.2294)
  spline S174 degree 3 poles (57.3352, -57.2294) (57.3352, -57.2558) (57.3617, -57.2294) (57.3352, -57.2294) knots 0 0 0 0 1 1 1 1
  line L194 (57.3352, -57.2294) -> (56.5679, -57.2294)
  line L195 (59.7429, -57.2294) -> (58.9756, -57.2294)
  spline S175 degree 3 poles (58.9756, -57.2294) (58.9492, -57.2294) (58.9756, -57.2558) (58.9756, -57.2294) knots 0 0 0 0 1 1 1 1
  line L196 (58.9756, -57.2294) -> (58.9756, -56.4885)
  spline S176 degree 3 poles (58.9756, -56.4885) (58.9756, -56.4621) (58.9492, -56.4885) (58.9756, -56.4885) knots 0 0 0 0 1 1 1 1
  line L197 (58.9756, -56.4885) -> (60.5102, -56.4885)
  spline S177 degree 3 poles (60.5102, -56.4885) (60.5367, -56.4885) (60.5102, -56.4621) (60.5102, -56.4885) knots 0 0 0 0 1 1 1 1
  line L198 (60.5102, -56.4885) -> (60.5102, -57.2294)
  spline S178 degree 3 poles (60.5102, -57.2294) (60.5102, -57.2558) (60.5367, -57.2294) (60.5102, -57.2294) knots 0 0 0 0 1 1 1 1
  line L199 (60.5102, -57.2294) -> (59.7429, -57.2294)
  line L200 (62.9179, -57.2294) -> (62.1506, -57.2294)
  spline S179 degree 3 poles (62.1506, -57.2294) (62.1242, -57.2294) (62.1506, -57.2558) (62.1506, -57.2294) knots 0 0 0 0 1 1 1 1
  line L201 (62.1506, -57.2294) -> (62.1506, -56.4885)
  spline S180 degree 3 poles (62.1506, -56.4885) (62.1506, -56.4621) (62.1242, -56.4885) (62.1506, -56.4885) knots 0 0 0 0 1 1 1 1
  line L202 (62.1506, -56.4885) -> (63.6852, -56.4885)
  spline S181 degree 3 poles (63.6852, -56.4885) (63.7117, -56.4885) (63.6852, -56.4621) (63.6852, -56.4885) knots 0 0 0 0 1 1 1 1
  line L203 (63.6852, -56.4885) -> (63.6852, -57.2294)
  spline S182 degree 3 poles (63.6852, -57.2294) (63.6852, -57.2558) (63.7117, -57.2294) (63.6852, -57.2294) knots 0 0 0 0 1 1 1 1
  line L204 (63.6852, -57.2294) -> (62.9179, -57.2294)
  line L205 (66.0929, -57.2294) -> (65.3256, -57.2294)
  spline S183 degree 3 poles (65.3256, -57.2294) (65.2992, -57.2294) (65.3256, -57.2558) (65.3256, -57.2294) knots 0 0 0 0 1 1 1 1
  line L206 (65.3256, -57.2294) -> (65.3256, -56.4885)
  spline S184 degree 3 poles (65.3256, -56.4885) (65.3256, -56.4621) (65.2992, -56.4885) (65.3256, -56.4885) knots 0 0 0 0 1 1 1 1
  line L207 (65.3256, -56.4885) -> (66.8602, -56.4885)
  spline S185 degree 3 poles (66.8602, -56.4885) (66.8867, -56.4885) (66.8602, -56.4621) (66.8602, -56.4885) knots 0 0 0 0 1 1 1 1
  line L208 (66.8602, -56.4885) -> (66.8602, -57.2294)
  spline S186 degree 3 poles (66.8602, -57.2294) (66.8602, -57.2558) (66.8867, -57.2294) (66.8602, -57.2294) knots 0 0 0 0 1 1 1 1
  line L209 (66.8602, -57.2294) -> (66.0929, -57.2294)
  line L210 (69.2679, -57.2294) -> (68.5006, -57.2294)
  spline S187 degree 3 poles (68.5006, -57.2294) (68.4742, -57.2294) (68.5006, -57.2558) (68.5006, -57.2294) knots 0 0 0 0 1 1 1 1
  line L211 (68.5006, -57.2294) -> (68.5006, -56.4885)
  spline S188 degree 3 poles (68.5006, -56.4885) (68.5006, -56.4621) (68.4742, -56.4885) (68.5006, -56.4885) knots 0 0 0 0 1 1 1 1
  line L212 (68.5006, -56.4885) -> (70.0352, -56.4885)
  spline S189 degree 3 poles (70.0352, -56.4885) (70.0617, -56.4885) (70.0352, -56.4621) (70.0352, -56.4885) knots 0 0 0 0 1 1 1 1
  line L213 (70.0352, -56.4885) -> (70.0352, -57.2294)
  spline S190 degree 3 poles (70.0352, -57.2294) (70.0352, -57.2558) (70.0617, -57.2294) (70.0352, -57.2294) knots 0 0 0 0 1 1 1 1
  line L214 (70.0352, -57.2294) -> (69.2679, -57.2294)
  line L215 (72.4429, -57.2294) -> (71.6756, -57.2294)
  spline S191 degree 3 poles (71.6756, -57.2294) (71.6492, -57.2294) (71.6756, -57.2558) (71.6756, -57.2294) knots 0 0 0 0 1 1 1 1
  line L216 (71.6756, -57.2294) -> (71.6756, -56.4885)
  spline S192 degree 3 poles (71.6756, -56.4885) (71.6756, -56.4621) (71.6492, -56.4885) (71.6756, -56.4885) knots 0 0 0 0 1 1 1 1
  line L217 (71.6756, -56.4885) -> (73.2102, -56.4885)
  spline S193 degree 3 poles (73.2102, -56.4885) (73.2367, -56.4885) (73.2102, -56.4621) (73.2102, -56.4885) knots 0 0 0 0 1 1 1 1
  line L218 (73.2102, -56.4885) -> (73.2102, -57.2294)
  spline S194 degree 3 poles (73.2102, -57.2294) (73.2102, -57.2558) (73.2367, -57.2294) (73.2102, -57.2294) knots 0 0 0 0 1 1 1 1
  line L219 (73.2102, -57.2294) -> (72.4429, -57.2294)
  line L220 (76.6434, -56.6272) -> (75.9021, -56.8259)
  spline S195 degree 3 poles (75.9021, -56.8259) (75.8767, -56.8328) (75.909, -56.8513) (75.9021, -56.8259) knots 0 0 0 0 1 1 1 1
  line L221 (75.9021, -56.8259) -> (75.7105, -56.1102)
  spline S196 degree 3 poles (75.7105, -56.1102) (75.7036, -56.0845) (75.6849, -56.1171) (75.7105, -56.1102) knots 0 0 0 0 1 1 1 1
  line L222 (75.7105, -56.1102) -> (77.1927, -55.713)
  spline S197 degree 3 poles (77.1927, -55.713) (77.2184, -55.7062) (77.1858, -55.6874) (77.1927, -55.713) knots 0 0 0 0 1 1 1 1
  line L223 (77.1927, -55.713) -> (77.3845, -56.4287)
  spline S198 degree 3 poles (77.3845, -56.4287) (77.3914, -56.4541) (77.4099, -56.4219) (77.3845, -56.4287) knots 0 0 0 0 1 1 1 1
  line L224 (77.3845, -56.4287) -> (76.6434, -56.6272)
  line L225 (80.7109, -54.279) -> (80.1682, -54.8214)
  spline S199 degree 3 poles (80.1682, -54.8214) (80.1494, -54.8402) (80.187, -54.8402) (80.1682, -54.8214) knots 0 0 0 0 1 1 1 1
  line L226 (80.1682, -54.8214) -> (79.6443, -54.2975)
  spline S200 degree 3 poles (79.6443, -54.2975) (79.6256, -54.279) (79.6256, -54.3163) (79.6443, -54.2975) knots 0 0 0 0 1 1 1 1
  line L227 (79.6443, -54.2975) -> (80.7294, -53.2125)
  spline S201 degree 3 poles (80.7294, -53.2125) (80.7482, -53.1937) (80.7109, -53.1937) (80.7294, -53.2125) knots 0 0 0 0 1 1 1 1
  line L228 (80.7294, -53.2125) -> (81.2533, -53.7363)
  spline S202 degree 3 poles (81.2533, -53.7363) (81.2721, -53.7551) (81.2721, -53.7176) (81.2533, -53.7363) knots 0 0 0 0 1 1 1 1
  line L229 (81.2533, -53.7363) -> (80.7109, -54.279)
  line L230 (83.0591, -50.2116) -> (82.8606, -50.9527)
  spline S203 degree 3 poles (82.8606, -50.9527) (82.8537, -50.9781) (82.886, -50.9595) (82.8606, -50.9527) knots 0 0 0 0 1 1 1 1
  line L231 (82.8606, -50.9527) -> (82.1449, -50.7608)
  spline S204 degree 3 poles (82.1449, -50.7608) (82.1193, -50.754) (82.138, -50.7865) (82.1449, -50.7608) knots 0 0 0 0 1 1 1 1
  line L232 (82.1449, -50.7608) -> (82.5421, -49.2786)
  spline S205 degree 3 poles (82.5421, -49.2786) (82.5489, -49.253) (82.5164, -49.2718) (82.5421, -49.2786) knots 0 0 0 0 1 1 1 1
  line L233 (82.5421, -49.2786) -> (83.2578, -49.4702)
  spline S206 degree 3 poles (83.2578, -49.4702) (83.2832, -49.4771) (83.2646, -49.4448) (83.2578, -49.4702) knots 0 0 0 0 1 1 1 1
  line L234 (83.2578, -49.4702) -> (83.0591, -50.2116)
  line L235 (83.6613, -45.2173) -> (83.6613, -45.9846)
  spline S207 degree 3 poles (83.6613, -45.9846) (83.6613, -46.011) (83.6877, -45.9846) (83.6613, -45.9846) knots 0 0 0 0 1 1 1 1
  line L236 (83.6613, -45.9846) -> (82.9204, -45.9846)
  spline S208 degree 3 poles (82.9204, -45.9846) (82.894, -45.9846) (82.9204, -46.011) (82.9204, -45.9846) knots 0 0 0 0 1 1 1 1
  line L237 (82.9204, -45.9846) -> (82.9204, -44.45)
  spline S209 degree 3 poles (82.9204, -44.45) (82.9204, -44.4235) (82.894, -44.45) (82.9204, -44.45) knots 0 0 0 0 1 1 1 1
  line L238 (82.9204, -44.45) -> (83.6613, -44.45)
  spline S210 degree 3 poles (83.6613, -44.45) (83.6877, -44.45) (83.6613, -44.4235) (83.6613, -44.45) knots 0 0 0 0 1 1 1 1
  line L239 (83.6613, -44.45) -> (83.6613, -45.2173)
  line L240 (45.1908, -58.4465) -> (46.7519, -58.4465)
  spline S211 degree 3 poles (46.7519, -58.4465) (46.7783, -58.4465) (46.7519, -58.42) (46.7519, -58.4465) knots 0 0 0 0 1 1 1 1
  line L241 (46.7519, -58.4465) -> (46.7519, -59.2138)
  spline S212 degree 3 poles (46.7519, -59.2138) (46.7519, -59.2283) (46.7638, -59.2402) (46.7783, -59.2402) knots 0 0 0 0 1 1 1 1
  line L242 (46.7783, -59.2402) -> (48.3658, -59.2402)
  spline S213 degree 3 poles (48.3658, -59.2402) (48.3804, -59.2402) (48.3923, -59.2283) (48.3923, -59.2138) knots 0 0 0 0 1 1 1 1
  line L243 (48.3923, -59.2138) -> (48.3923, -58.4465)
  spline S214 degree 3 poles (48.3923, -58.4465) (48.3923, -58.42) (48.3658, -58.4465) (48.3923, -58.4465) knots 0 0 0 0 1 1 1 1
  line L244 (48.3923, -58.4465) -> (49.9269, -58.4465)
  spline S215 degree 3 poles (49.9269, -58.4465) (49.9533, -58.4465) (49.9269, -58.42) (49.9269, -58.4465) knots 0 0 0 0 1 1 1 1
  line L245 (49.9269, -58.4465) -> (49.9269, -59.2138)
  spline S216 degree 3 poles (49.9269, -59.2138) (49.9269, -59.2283) (49.9388, -59.2402) (49.9533, -59.2402) knots 0 0 0 0 1 1 1 1
  line L246 (49.9533, -59.2402) -> (51.5408, -59.2402)
  spline S217 degree 3 poles (51.5408, -59.2402) (51.5554, -59.2402) (51.5673, -59.2283) (51.5673, -59.2138) knots 0 0 0 0 1 1 1 1
  line L247 (51.5673, -59.2138) -> (51.5673, -58.4465)
  spline S218 degree 3 poles (51.5673, -58.4465) (51.5673, -58.42) (51.5408, -58.4465) (51.5673, -58.4465) knots 0 0 0 0 1 1 1 1
  line L248 (51.5673, -58.4465) -> (53.1019, -58.4465)
  spline S219 degree 3 poles (53.1019, -58.4465) (53.1283, -58.4465) (53.1019, -58.42) (53.1019, -58.4465) knots 0 0 0 0 1 1 1 1
  line L249 (53.1019, -58.4465) -> (53.1019, -59.2138)
  spline S220 degree 3 poles (53.1019, -59.2138) (53.1019, -59.2283) (53.1138, -59.2402) (53.1283, -59.2402) knots 0 0 0 0 1 1 1 1
  line L250 (53.1283, -59.2402) -> (54.7158, -59.2402)
  spline S221 degree 3 poles (54.7158, -59.2402) (54.7304, -59.2402) (54.7423, -59.2283) (54.7423, -59.2138) knots 0 0 0 0 1 1 1 1
  line L251 (54.7423, -59.2138) -> (54.7423, -58.4465)
  spline S222 degree 3 poles (54.7423, -58.4465) (54.7423, -58.42) (54.7158, -58.4465) (54.7423, -58.4465) knots 0 0 0 0 1 1 1 1
  line L252 (54.7423, -58.4465) -> (56.2769, -58.4465)
  spline S223 degree 3 poles (56.2769, -58.4465) (56.3033, -58.4465) (56.2769, -58.42) (56.2769, -58.4465) knots 0 0 0 0 1 1 1 1
  line L253 (56.2769, -58.4465) -> (56.2769, -59.2138)
  spline S224 degree 3 poles (56.2769, -59.2138) (56.2769, -59.2283) (56.2888, -59.2402) (56.3033, -59.2402) knots 0 0 0 0 1 1 1 1
  line L254 (56.3033, -59.2402) -> (57.8908, -59.2402)
  spline S225 degree 3 poles (57.8908, -59.2402) (57.9054, -59.2402) (57.9173, -59.2283) (57.9173, -59.2138) knots 0 0 0 0 1 1 1 1
  line L255 (57.9173, -59.2138) -> (57.9173, -58.4465)
  spline S226 degree 3 poles (57.9173, -58.4465) (57.9173, -58.42) (57.8908, -58.4465) (57.9173, -58.4465) knots 0 0 0 0 1 1 1 1
  line L256 (57.9173, -58.4465) -> (59.4519, -58.4465)
  spline S227 degree 3 poles (59.4519, -58.4465) (59.4783, -58.4465) (59.4519, -58.42) (59.4519, -58.4465) knots 0 0 0 0 1 1 1 1
  line L257 (59.4519, -58.4465) -> (59.4519, -59.2138)
  spline S228 degree 3 poles (59.4519, -59.2138) (59.4519, -59.2283) (59.4638, -59.2402) (59.4783, -59.2402) knots 0 0 0 0 1 1 1 1
  line L258 (59.4783, -59.2402) -> (61.0658, -59.2402)
  spline S229 degree 3 poles (61.0658, -59.2402) (61.0804, -59.2402) (61.0923, -59.2283) (61.0923, -59.2138) knots 0 0 0 0 1 1 1 1
  line L259 (61.0923, -59.2138) -> (61.0923, -58.4465)
  spline S230 degree 3 poles (61.0923, -58.4465) (61.0923, -58.42) (61.0658, -58.4465) (61.0923, -58.4465) knots 0 0 0 0 1 1 1 1
  line L260 (61.0923, -58.4465) -> (62.6269, -58.4465)
  spline S231 degree 3 poles (62.6269, -58.4465) (62.6533, -58.4465) (62.6269, -58.42) (62.6269, -58.4465) knots 0 0 0 0 1 1 1 1
  line L261 (62.6269, -58.4465) -> (62.6269, -59.2138)
  spline S232 degree 3 poles (62.6269, -59.2138) (62.6269, -59.2283) (62.6388, -59.2402) (62.6533, -59.2402) knots 0 0 0 0 1 1 1 1
  line L262 (62.6533, -59.2402) -> (64.2408, -59.2402)
  spline S233 degree 3 poles (64.2408, -59.2402) (64.2554, -59.2402) (64.2673, -59.2283) (64.2673, -59.2138) knots 0 0 0 0 1 1 1 1
  line L263 (64.2673, -59.2138) -> (64.2673, -58.4465)
  spline S234 degree 3 poles (64.2673, -58.4465) (64.2673, -58.42) (64.2408, -58.4465) (64.2673, -58.4465) knots 0 0 0 0 1 1 1 1
  line L264 (64.2673, -58.4465) -> (65.8019, -58.4465)
  spline S235 degree 3 poles (65.8019, -58.4465) (65.8283, -58.4465) (65.8019, -58.42) (65.8019, -58.4465) knots 0 0 0 0 1 1 1 1
  line L265 (65.8019, -58.4465) -> (65.8019, -59.2138)
  spline S236 degree 3 poles (65.8019, -59.2138) (65.8019, -59.2283) (65.8138, -59.2402) (65.8283, -59.2402) knots 0 0 0 0 1 1 1 1
  line L266 (65.8283, -59.2402) -> (67.4158, -59.2402)
  spline S237 degree 3 poles (67.4158, -59.2402) (67.4304, -59.2402) (67.4423, -59.2283) (67.4423, -59.2138) knots 0 0 0 0 1 1 1 1
  line L267 (67.4423, -59.2138) -> (67.4423, -58.4465)
  spline S238 degree 3 poles (67.4423, -58.4465) (67.4423, -58.42) (67.4158, -58.4465) (67.4423, -58.4465) knots 0 0 0 0 1 1 1 1
  line L268 (67.4423, -58.4465) -> (68.9769, -58.4465)
  spline S239 degree 3 poles (68.9769, -58.4465) (69.0033, -58.4465) (68.9769, -58.42) (68.9769, -58.4465) knots 0 0 0 0 1 1 1 1
  line L269 (68.9769, -58.4465) -> (68.9769, -59.2138)
  spline S240 degree 3 poles (68.9769, -59.2138) (68.9769, -59.2283) (68.9888, -59.2402) (69.0033, -59.2402) knots 0 0 0 0 1 1 1 1
  line L270 (69.0033, -59.2402) -> (70.5908, -59.2402)
  spline S241 degree 3 poles (70.5908, -59.2402) (70.6054, -59.2402) (70.6173, -59.2283) (70.6173, -59.2138) knots 0 0 0 0 1 1 1 1
  line L271 (70.6173, -59.2138) -> (70.6173, -58.4465)
  spline S242 degree 3 poles (70.6173, -58.4465) (70.6173, -58.42) (70.5908, -58.4465) (70.6173, -58.4465) knots 0 0 0 0 1 1 1 1
  line L272 (70.6173, -58.4465) -> (72.1519, -58.4465)
  spline S243 degree 3 poles (72.1519, -58.4465) (72.1783, -58.4465) (72.1519, -58.42) (72.1519, -58.4465) knots 0 0 0 0 1 1 1 1
  line L273 (72.1519, -58.4465) -> (72.1519, -59.2138)
  spline S244 degree 3 poles (72.1519, -59.2138) (72.1519, -59.2283) (72.1638, -59.2402) (72.1783, -59.2402) knots 0 0 0 0 1 1 1 1
  line L274 (72.1783, -59.2402) -> (73.7658, -59.2402)
  spline S245 degree 3 poles (73.7658, -59.2402) (73.7804, -59.2402) (73.7923, -59.2283) (73.7923, -59.2138) knots 0 0 0 0 1 1 1 1
  line L275 (73.7923, -59.2138) -> (73.7923, -58.4465)
  spline S246 degree 3 poles (73.7923, -58.4465) (73.7923, -58.42) (73.7658, -58.4465) (73.7923, -58.4465) knots 0 0 0 0 1 1 1 1
  line L276 (73.7923, -58.4465) -> (75.3269, -58.4465)
  spline S247 degree 3 poles (75.3269, -58.4465) (75.3533, -58.4465) (75.3269, -58.42) (75.3269, -58.4465) knots 0 0 0 0 1 1 1 1
  line L277 (75.3269, -58.4465) -> (75.3269, -59.2138)
  spline S248 degree 3 poles (75.3269, -59.2138) (75.3269, -59.2283) (75.3388, -59.2402) (75.3533, -59.2402) knots 0 0 0 0 1 1 1 1
  line L278 (75.3533, -59.2402) -> (76.9408, -59.2402)
  spline S249 degree 3 poles (76.9408, -59.2402) (76.9554, -59.2402) (76.9673, -59.2283) (76.9673, -59.2138) knots 0 0 0 0 1 1 1 1
  line L279 (76.9673, -59.2138) -> (76.9673, -58.4465)
  spline S250 degree 3 poles (76.9673, -58.4465) (76.9673, -58.42) (76.9408, -58.4465) (76.9673, -58.4465) knots 0 0 0 0 1 1 1 1
  line L280 (76.9673, -58.4465) -> (78.5019, -58.4465)
  spline S251 degree 3 poles (78.5019, -58.4465) (78.5283, -58.4465) (78.5019, -58.42) (78.5019, -58.4465) knots 0 0 0 0 1 1 1 1
  line L281 (78.5019, -58.4465) -> (78.5019, -59.2138)
  spline S252 degree 3 poles (78.5019, -59.2138) (78.5019, -59.2283) (78.5138, -59.2402) (78.5283, -59.2402) knots 0 0 0 0 1 1 1 1
  line L282 (78.5283, -59.2402) -> (80.1158, -59.2402)
  spline S253 degree 3 poles (80.1158, -59.2402) (80.1304, -59.2402) (80.1423, -59.2283) (80.1423, -59.2138) knots 0 0 0 0 1 1 1 1
  line L283 (80.1423, -59.2138) -> (80.1423, -58.4465)
  spline S254 degree 3 poles (80.1423, -58.4465) (80.1423, -58.42) (80.1158, -58.4465) (80.1423, -58.4465) knots 0 0 0 0 1 1 1 1
  line L284 (80.1423, -58.4465) -> (81.6769, -58.4465)
  spline S255 degree 3 poles (81.6769, -58.4465) (81.7033, -58.4465) (81.6769, -58.42) (81.6769, -58.4465) knots 0 0 0 0 1 1 1 1
  line L285 (81.6769, -58.4465) -> (81.6769, -59.2138)
  spline S256 degree 3 poles (81.6769, -59.2138) (81.6769, -59.2283) (81.6888, -59.2402) (81.7033, -59.2402) knots 0 0 0 0 1 1 1 1
  line L286 (81.7033, -59.2402) -> (83.2908, -59.2402)
  spline S257 degree 3 poles (83.2908, -59.2402) (83.3054, -59.2402) (83.3173, -59.2283) (83.3173, -59.2138) knots 0 0 0 0 1 1 1 1
  line L287 (83.3173, -59.2138) -> (83.3173, -58.4465)
  spline S258 degree 3 poles (83.3173, -58.4465) (83.3173, -58.42) (83.2908, -58.4465) (83.3173, -58.4465) knots 0 0 0 0 1 1 1 1
  line L288 (83.3173, -58.4465) -> (84.8783, -58.4465)
  spline S259 degree 3 poles (84.8783, -58.4465) (84.8929, -58.4465) (84.9048, -58.4346) (84.9048, -58.42) knots 0 0 0 0 1 1 1 1
  line L289 (84.9048, -58.42) -> (84.9048, -57.6527)
  spline S260 degree 3 poles (84.9048, -57.6527) (84.9048, -57.6263) (84.8783, -57.6527) (84.9048, -57.6527) knots 0 0 0 0 1 1 1 1
  line L290 (84.9048, -57.6527) -> (85.6721, -57.6527)